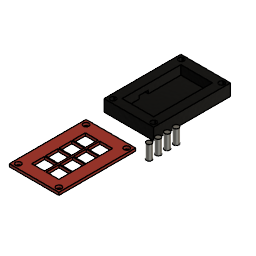
noahs-macropad (Autodesk Fusion 360 design; units mm, degrees)
part number: 2026-02-17-16-46-34-491
Autodesk Fusion 360 part; units mm, degrees
sketch "Sketch1" plane through (0, 0, 0) normal (0, 0, 1) x (1, 0, 0)
box "BoxPrimitive2" add length 85.12 width 54.94 height 3 placed x (0, 1, 0) y (-1, 0, 0) z (0, 0, 1) at (54.94, 0, 0) makes body 1
box "BoxPrimitive3" add length 85.12 width 10 height 10 placed x (0, 1, 0) y (-1, 0, 0) z (0, 0, 1) at (10, 0, 3) bodies 1
box "BoxPrimitive4" add length 10 width 44.94 height 10 placed x (0, 1, 0) y (-1, 0, 0) z (0, 0, 1) at (54.94, 0, 3) bodies 1
box "BoxPrimitive5" add length 75.12 width 10 height 10 placed x (0, -1, 0) y (1, 0, 0) z (0, 0, 1) at (44.94, 85.12, 3) bodies 1
box "BoxPrimitive6" add length 10 width 34.94 height 10 placed x (0, -1, 0) y (1, 0, 0) z (0, 0, 1) at (10, 85.12, 3) bodies 1
sketch "Sketch8" plane through (10, 0, 0) normal (1, 0, 0) x (0, 1, 0)
  line L0 (75.12, 3) -> (75.12, 13)
  line L1 (75.12, 13) -> (10, 13)
  line L2 (10, 13) -> (10, 3)
  line L3 (10, 3) -> (75.12, 3)
  line L4 (29, 3) -> (39, 3)
  line L5 (39, 3) -> (39, 6.5245)
  line L6 (39, 6.5245) -> (29, 6.5245)
  line L7 (29, 6.5245) -> (29, 3)
  dimension "d39" = 10
  constraint horizontal L4
  constraint vertical L5
  constraint horizontal L6
  constraint vertical L7
  constraint coincident L3 L4.start
  measures "d39" distance of L4.start L4.end
extrude "Extrude1" cut sketch "Sketch8" against normal blind 10 contours L3 L4 L5 L6 L7 bodies 1
hole "Hole1" at (5.1129, 4.8805, 13) direction (0, 0, -1) diameter 6 depth 10 tip angle 180 bodies 1
hole "Hole2" at (5.2749, 80.4444, 13) direction (0, 0, -1) diameter 6 depth 10 tip angle 180 bodies 1
hole "Hole3" at (50.3076, 4.7995, 13) direction (0, 0, -1) diameter 6 depth 10 tip angle 180 bodies 1
hole "Hole4" at (50.3076, 80.2014, 13) direction (0, 0, -1) diameter 6 depth 10 tip angle 180 bodies 1
box "BoxPrimitive7" add length 85.12 width 54.94 height 3 placed x (0, 1, 0) y (-1, 0, 0) z (0, 0, 1) at (54.94, -105, 0) separate body makes body 2
sketch "Sketch10" plane through (0, 0, 3) normal (0, 0, 1) x (-1, 0, 0)
  line L0 (-54.94, 19.88) -> (0, 19.88)
  line L1 (0, 19.88) -> (0, 105)
  line L2 (0, 105) -> (-54.94, 105)
  line L3 (-54.94, 105) -> (-54.94, 19.88)
  line L4 (-10, 95) -> (-45, 95)
  line L5 (-45, 95) -> (-45, 25)
  line L6 (-26.525, 92.475) -> (-12.525, 92.475)
  line L7 (-12.525, 92.475) -> (-12.525, 78.475)
  line L8 (-12.525, 78.475) -> (-26.525, 78.475)
  line L9 (-26.525, 78.475) -> (-26.525, 92.475)
  line L10 (-45, 95) -> (-45, 85.475)
  line L11 (-28.475, 78.475) -> (-42.475, 78.475)
  line L12 (-42.475, 78.475) -> (-42.475, 92.475)
  line L13 (-42.475, 92.475) -> (-28.475, 92.475)
  line L14 (-28.475, 92.475) -> (-28.475, 78.475)
  dimension "d75" = 14
  dimension "d76" = 14
  dimension "d78" = 9.525
  dimension "d82" = 14
  dimension "d83" = 14
  constraint horizontal L4
  constraint perpendicular L4 L5
  constraint horizontal L6
  constraint vertical L7
  constraint horizontal L8
  constraint vertical L9
  constraint perpendicular L4 L10
  constraint horizontal L11
  constraint vertical L12
  constraint horizontal L13
  constraint vertical L14
  measures "d75" distance of L6.start L6.end
  measures "d76" distance of L6.start L8.end
  measures "d78" distance of L4.end L10.end
  measures "d82" distance of L11.start L11.end
  measures "d83" distance of L11.start L13.end
extrude "Extrude2" cut sketch "Sketch10" against normal blind 3 contours L6 L7 L8 L9 | L11 L12 L13 L14 bodies 2
sketch "Sketch11" plane through (0, 0, 3) normal (0, 0, 1) x (-1, 0, 0)
  line L0 (-12.525, 92.475) -> (-12.525, 78.475)
  line L1 (-12.525, 78.475) -> (-26.525, 78.475)
  line L2 (-26.525, 92.475) -> (-12.525, 92.475)
  line L3 (-42.475, 78.475) -> (-42.475, 92.475)
  line L4 (-42.475, 92.475) -> (-28.475, 92.475)
  line L5 (-28.475, 78.475) -> (-42.475, 78.475)
  line L6 (-54.94, 19.88) -> (0, 19.88)
  line L7 (0, 19.88) -> (0, 105)
  line L8 (0, 105) -> (-54.94, 105)
  line L9 (-54.94, 105) -> (-54.94, 19.88)
  line L10 (-45, 95) -> (-44.94, 29.88)
  line L11 (-10, 29.88) -> (-44.94, 29.88)
  line L12 (-35.475, 70.385) -> (-42.475, 70.385)
  line L13 (-42.475, 77.385) -> (-28.475, 77.385)
  line L14 (-28.475, 77.385) -> (-28.475, 63.385)
  line L15 (-28.475, 63.385) -> (-42.475, 63.385)
  line L16 (-42.475, 63.385) -> (-42.475, 77.385)
  line L17 (-42.475, 62.295) -> (-28.475, 62.295)
  line L18 (-28.475, 62.295) -> (-28.475, 48.295)
  line L19 (-28.475, 48.295) -> (-42.475, 48.295)
  line L20 (-42.475, 48.295) -> (-42.475, 62.295)
  line L21 (-42.475, 47.205) -> (-28.475, 47.205)
  line L22 (-28.475, 47.205) -> (-28.475, 33.205)
  line L23 (-28.475, 33.205) -> (-42.475, 33.205)
  line L24 (-42.475, 33.205) -> (-42.475, 47.205)
  line L25 (-26.525, 78.475) -> (-12.525, 78.475)
  line L26 (-26.525, 78.475) -> (-19.525, 78.475)
  line L27 (-12.525, 63.385) -> (-26.525, 63.385)
  line L28 (-26.525, 63.385) -> (-26.525, 77.385)
  line L29 (-26.525, 77.385) -> (-12.525, 77.385)
  line L30 (-12.525, 77.385) -> (-12.525, 63.385)
  line L31 (-26.525, 62.295) -> (-12.525, 62.295)
  line L32 (-12.525, 62.295) -> (-12.525, 48.295)
  line L33 (-12.525, 48.295) -> (-26.525, 48.295)
  line L34 (-26.525, 48.295) -> (-26.525, 62.295)
  line L35 (-26.525, 47.205) -> (-12.525, 47.205)
  line L36 (-12.525, 47.205) -> (-12.525, 33.205)
  line L37 (-12.525, 33.205) -> (-26.525, 33.205)
  line L38 (-26.525, 33.205) -> (-26.525, 47.205)
  dimension "d89" = 7
  dimension "d90" = 14
  dimension "d91" = 14
  dimension "d95" = 14
  dimension "d96" = 14
  dimension "d100" = 14
  dimension "d101" = 14
  dimension "d103" = 7
  dimension "d107" = 14
  dimension "d108" = 14
  dimension "d111" = 14
  dimension "d112" = 14
  dimension "d116" = 14
  dimension "d117" = 14
  constraint horizontal L11
  constraint horizontal L13
  constraint vertical L14
  constraint horizontal L15
  constraint vertical L16
  constraint horizontal L17
  constraint vertical L18
  constraint horizontal L19
  constraint vertical L20
  constraint horizontal L21
  constraint vertical L22
  constraint horizontal L23
  constraint vertical L24
  constraint coincident L1.end L25.start
  constraint coincident L0.end L1.start
  constraint horizontal L27
  constraint vertical L28
  constraint horizontal L29
  constraint vertical L30
  constraint horizontal L31
  constraint vertical L32
  constraint horizontal L33
  constraint vertical L34
  constraint horizontal L35
  constraint vertical L36
  constraint horizontal L37
  constraint vertical L38
  measures "d89" distance of L12.end L13.start
  measures "d90" distance of L13.start L13.end
  measures "d91" distance of L13.start L15.end
  measures "d95" distance of L17.start L17.end
  measures "d96" distance of L17.start L19.end
  measures "d100" distance of L21.start L21.end
  measures "d101" distance of L21.start L23.end
  measures "d103" distance of L1.end L26.end
  measures "d107" distance of L27.start L27.end
  measures "d108" distance of L27.start L29.end
  measures "d111" distance of L31.start L31.end
  measures "d112" distance of L31.start L33.end
  measures "d116" distance of L35.start L35.end
  measures "d117" distance of L35.start L37.end
extrude "Extrude3" cut sketch "Sketch11" against normal blind 3 contours L13 L14 L15 L16 | L17 L18 L19 L20 | L21 L22 L23 L24 | L27 L28 L29 L30 | L31 L32 L33 L34 | L35 L36 L37 L38 bodies 2
hole "Hole5" at (5.0857, -100.0691, 3) direction (0, 0, -1) diameter 6 depth 10 tip angle 180 bodies 2
hole "Hole6" at (5.0901, -24.9289, 3) direction (0, 0, -1) diameter 6 depth 10 tip angle 180 bodies 2
hole "Hole7" at (50.0503, -24.8776, 3) direction (0, 0, -1) diameter 6 depth 10 tip angle 180 bodies 2
hole "Hole8" at (50.0073, -99.9715, 3) direction (0, 0, -1) diameter 6 depth 10 tip angle 180 bodies 2
cylinder "CylinderPrimitive4" add diameter 6 height 16 placed x (1, 0, 0) y (0, 1, 0) z (0, 0, 1) at (70, 0, 0) separate body makes body 3
copy_body "CopyPasteBodies1" bodies 3 makes body 4
move_body "Move1" bodies 4 to x (1, 0, 0) y (0, 1, 0) z (0, 0, 1) at (0, 10, 0)
copy_body "CopyPasteBodies2" bodies 3 makes body 5
move_body "Move2" bodies 5 to x (1, 0, 0) y (0, 1, 0) z (0, 0, 1) at (0, -10, 0)
copy_body "CopyPasteBodies3" bodies 3 makes body 6
move_body "Move3" bodies 6 to x (1, 0, 0) y (0, 1, 0) z (0, 0, 1) at (0, -20, 0)
